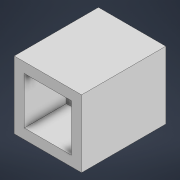
# Autodesk Inventor part: Clip_MarkerHolderV1
Saved by Autodesk Inventor 2022 (Build 260153000, 153)
## iProperties
Created: 2023-05-06
Part Number: Clip_MarkerHolderV1
Material: Generic
Document SubType Name: Modeling
Designer: Karl Spiteri
Density: 1 g/cm^3
Appearance: Default
Author: Karl Spiteri
Autodesk Inventor part; units mm, degrees
ref_plane "YZ Plane" through (0, 0, 0) normal (1, 0, 0) x (0, 1, 0)
ref_plane "XZ Plane" through (0, 0, 0) normal (0, 1, 0) x (-1, 0, 0)
ref_plane "XY Plane" through (0, 0, 0) normal (0, 0, 1) x (1, 0, 0)
sketch "Sketch4" plane through (0, 0, 0) normal (0, 0, 1) x (1, 0, 0)
  line L0 (0, 0) -> (-8, 0)
  line L1 (-8, 0) -> (-8, 8)
  line L2 (-8, 8) -> (0, 8)
  line L3 (0, 8) -> (0, 0)
  dimension "d30" = 8
  dimension "d31" = 8
  constraints: 8 end point, 2 parallel, 1 horizontal, 1 perpendicular
  measures "d30" distance of L1.end L2.end
  measures "d31" distance of L0.end L1.end
extrude "Extrusion6" add sketch "Sketch4" along normal blind 10
sketch "Sketch6" plane through (0, 0, 10) normal (0, 0, 1) x (1, 0, 0)
  line L0 (-4, 4) -> (-6.8, 4)
  line L1 (-6.8, 4) -> (-6.8, 6.8)
  line L2 (-6.8, 6.8) -> (-4, 6.8)
  line L3 (-4, 6.8) -> (-4, 4)
  line L4 (-6.8, 6.8) -> (-1.2, 6.8)
  line L5 (-1.2, 6.8) -> (-1.2, 1.2)
  line L6 (-1.2, 1.2) -> (-6.8, 1.2)
  line L7 (-6.8, 1.2) -> (-6.8, 6.8)
  point P0 (0, 0)
  dimension "d40" = 2.8
  dimension "d41" = 2.8
  dimension "d42" = 5.6
  dimension "d43" = 5.6
  constraints: 16 end point, 4 parallel, 2 horizontal, 2 perpendicular
  measures "d40" distance of L1.end L2.end
  measures "d41" distance of L0.end L1.end
  measures "d42" distance of L5.end L6.end
  measures "d43" distance of L4.end L5.end
extrude "Extrusion8" cut sketch "Sketch6" against normal blind 5
body "Solid2"
